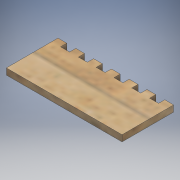
# Autodesk Inventor part: Side Support
Saved by Autodesk Inventor 2017 (Build 210142000, 142)
## iProperties
Created: 2017-05-02
Part Number: Side Support
Material: Generic
Document SubType Name: Modeling
Designer: Parshant Bombhi
Density: 1 g/cm^3
Appearance: Natural Maple - Glossy Dark Tint
Author: Parshant Bombhi
Autodesk Inventor part; units mm, degrees
ref_plane "YZ Plane" through (0, 0, 0) normal (1, 0, 0) x (0, 1, 0)
ref_plane "XZ Plane" through (0, 0, 0) normal (0, 1, 0) x (-1, 0, 0)
ref_plane "XY Plane" through (0, 0, 0) normal (0, 0, 1) x (1, 0, 0)
sketch "Sketch1" plane through (0, 0, 0) normal (0, 0, 1) x (1, 0, 0)
  line L0 (0, 0) -> (130, 0)
  line L1 (0, 58) -> (0, 0)
  line L2 (0, 58) -> (10, 58)
  line L3 (10, 51) -> (20, 51)
  line L4 (20, 51) -> (20, 58)
  line L5 (10, 51) -> (10, 58)
  line L6 (30, 58) -> (30, 51)
  line L7 (30, 51) -> (40, 51)
  line L8 (40, 51) -> (40, 58)
  line L9 (50, 58) -> (50, 51)
  line L10 (50, 51) -> (60, 51)
  line L11 (10, 58) -> (0, 58)
  line L12 (20, 58) -> (30, 58)
  line L13 (40, 58) -> (50, 58)
  line L14 (60, 51) -> (60, 58)
  line L15 (60, 58) -> (70, 58)
  line L16 (70, 58) -> (70, 51)
  line L17 (70, 51) -> (80, 51)
  line L18 (80, 51) -> (80, 58)
  line L19 (80, 58) -> (90, 58)
  line L20 (90, 58) -> (90, 51)
  line L21 (90, 51) -> (100, 51)
  line L22 (100, 51) -> (100, 58)
  line L23 (100, 58) -> (110, 58)
  line L24 (110, 58) -> (110, 51)
  line L25 (110, 51) -> (120, 51)
  line L26 (120, 51) -> (120, 58)
  line L27 (120, 58) -> (130, 58)
  line L28 (130, 58) -> (130, 51)
  line L29 (130, 51) -> (130, 51)
  line L30 (130, 51) -> (130, 0)
  dimension "Total_Width" = 130
  dimension "Teeth_Width" = 10
  dimension "Material_Thickness" = 7
  dimension "d4" = 10
  dimension "d5" = 10
  dimension "d6" = 10
  dimension "d9" = 10
  dimension "d12" = 10
  dimension "d13" = 10
  dimension "d14" = 10
  dimension "d15" = 10
  dimension "d16" = 10
  dimension "d17" = 10
  dimension "d18" = 10
  dimension "d19" = 10
  dimension "Total_Height" = 58
  constraints: 62 end point, 15 perpendicular, 12 point on line, 3 vertical, 2 horizontal, 2 parallel, 1 collinear
  measures "Total_Width" distance of L0.start L0.end
  measures "Teeth_Width" distance of L2.end L1.start
  measures "Material_Thickness" distance of L3.start L2.end
  measures "d4" distance of L3.start L3.end
  measures "d5" distance of L6.start L4.end
  measures "d6" distance of L6.end L7.end
  measures "d9" distance of L9.end L10.end
  measures "d12" distance of L8.end L9.start
  measures "d13" distance of L14.end L15.end
  measures "d14" distance of L16.end L17.end
  measures "d15" distance of L18.end L19.end
  measures "d16" distance of L20.end L21.end
  measures "d17" distance of L22.end L23.end
  measures "d18" distance of L24.end L25.end
  measures "d19" distance of L26.end L27.end
  measures "Total_Height" distance of L1.start L0.start
extrude "Extrusion1" add sketch "Sketch1" along normal blind 7
equation "\"d4\" = Teeth_Width"
equation "\"d5\" = Teeth_Width"
equation "\"d6\" = Teeth_Width"
equation "\"d9\" = Teeth_Width"
equation "\"d12\" = Teeth_Width"
equation "\"d13\" = Teeth_Width"
equation "\"d14\" = Teeth_Width"
equation "\"d15\" = Teeth_Width"
equation "\"d16\" = Teeth_Width"
equation "\"d17\" = Teeth_Width"
equation "\"d18\" = Teeth_Width"
equation "\"d19\" = Teeth_Width"
equation "\"d20\" = Material_Thickness"
body "Solid1"
